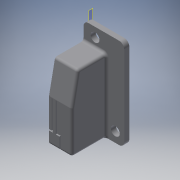
# Autodesk Inventor part: motorBracket_R
Saved by Autodesk Inventor 2016 (Build 200138000, 138)
## iProperties
Created: 2016-09-24
Part Number: motorBracket_R
Material: Generic
Document SubType Name: Modeling
Designer: benja
Density: 1 g/cm^3
Appearance: Default
Author: benja
Autodesk Inventor part; units mm, degrees
ref_plane "YZ Plane" through (0, 0, 0) normal (1, 0, 0) x (0, 1, 0)
ref_plane "XZ Plane" through (0, 0, 0) normal (0, 1, 0) x (-1, 0, 0)
ref_plane "XY Plane" through (0, 0, 0) normal (0, 0, 1) x (1, 0, 0)
ref_plane "Work Plane1" through (29.8157, -13.9206, -3.5875) normal (-1, 0, 0) x (0, -1, 0)
sketch "Sketch1" plane through (29.8157, -13.9206, -3.5875) normal (-1, 0, 0) x (0, -1, 0)
  line L0 (36.0555, 15.1875) -> (19.6981, 15.1875)
  line L1 (7.4278, 14.773) -> (19.5, 17.1875)
  line L2 (19.5, 17.1875) -> (36.0555, 17.1875)
  line L3 (36.0555, 17.1875) -> (36.0555, 15.1875)
  line L4 (0, 0) -> (36.0555, 0) projected
  line L5 (36.0555, 0) -> (36.0555, 1.5875) projected
  line L6 (0, 1.5875) -> (36.0555, 1.5875) projected
  line L7 (0, 0) -> (0, 1.5875) projected
  line L8 (37.8978, 2.9875) -> (37.8978, 4.6582) projected
  line L9 (19.6981, 15.1875) -> (9.4278, 13.1334)
  line L10 (9.4278, 13.1334) -> (9.4278, 2.5875)
  line L11 (9.4278, 2.5875) -> (36.0555, 2.5875)
  line L12 (36.0555, 2.5875) -> (36.0555, 1.5875)
  line L13 (0.4278, 3.5875) -> (7.4278, 3.5875)
  line L14 (7.4278, 3.5875) -> (7.4278, 14.773)
  arc A0 (20.8375, 9.9921) -> (19.4853, 10.9049) centre (20.7278, 11.2875) ccw projected
  arc A1 (19.4853, 10.9049) -> (20.8375, 9.9921) centre (18.0278, 7.2875) ccw projected
  circle A2 centre (15.9478, 12.4775) radius 0.925 projected
  circle A3 centre (12.5278, 5.6875) radius 0.5 projected
  circle A4 centre (30.6778, 13.1375) radius 0.5 projected
  line L15 (13.7278, 4.0975) -> (14.9378, 2.8875) projected
  line L16 (14.9378, 2.8875) -> (21.8778, 2.8875) projected
  line L17 (21.8778, 2.8875) -> (23.7478, 4.7575) projected
  line L18 (23.7478, 4.7575) -> (28.3978, 4.7575) projected
  line L19 (28.3978, 4.7575) -> (28.3978, 11.2875) projected
  line L20 (28.3978, 11.2875) -> (32.9778, 11.2875) projected
  line L21 (32.9778, 11.2875) -> (32.9778, 14.8875) projected
  line L22 (32.9778, 14.8875) -> (19.7278, 14.8875) projected
  line L23 (19.7278, 14.8875) -> (9.7278, 12.8875) projected
  line L24 (9.7278, 6.0975) -> (9.7278, 12.8875) projected
  line L25 (11.7278, 4.0975) -> (9.7278, 6.0975) projected
  line L26 (13.7278, 4.0975) -> (11.7278, 4.0975) projected
  circle A5 centre (27.3778, 12.9875) radius 0.925 projected
  line L27 (36.0555, 1.5875) -> (0, 1.5875)
  line L28 (0.4278, 3.5875) -> (0.4278, 1.5875)
  point P0 (-13.9206, 3.5875)
  dimension "d2" = 2
  dimension "d3" = 0.3
  dimension "d4" = 0.3
  dimension "d5" = 0.3
  dimension "d6" = 0.3
  dimension "d7" = 2
  dimension "d8" = 2
  dimension "d10" = 2
  dimension "d37" = 7
  constraints: 26 end point, 5 perpendicular, 1 collinear, 1 parallel, 1 point on line, 1 vertical
  measures "d2" distance between parallel lines of L2 L0
  measures "d3" distance between parallel lines of L11 L16
  measures "d4" distance between parallel lines of L10 L24
  measures "d5" distance between parallel lines of L23 L9
  measures "d6" distance between parallel lines of L22 L0
  measures "d7" distance between parallel lines of L6 L13
  measures "d8" distance between parallel lines of L14 L10
  measures "d10" distance between parallel lines of L9 L1
  measures "d37" distance between parallel lines of L14 L28
extrude "Extrusion1" add sketch "Sketch1" against normal blind 7.05 contours L0 L9 L10 L11 L12 L6 L28 L13 L14 L1 L2 L3
sketch "Sketch2" plane through (36.8657, -13.9206, -3.5875) normal (1, 0, 0) x (0, 0, -1)
  line L0 (-17.1875, -36.0555) -> (-15.1875, -36.0555) projected
  line L1 (-15.1875, -36.0555) -> (-15.1875, -19.6981) projected
  line L2 (-15.1875, -19.6981) -> (-13.1334, -9.4278) projected
  line L3 (-13.1334, -9.4278) -> (-2.5875, -9.4278) projected
  line L4 (-2.5875, -9.4278) -> (-2.5875, -36.0555) projected
  line L5 (-2.5875, -36.0555) -> (-1.5875, -36.0555) projected
  line L6 (-1.5875, -36.0555) -> (-1.5875, -0.4278) projected
  line L7 (-3.5875, -0.4278) -> (-3.5875, -7.4278) projected
  line L8 (-3.5875, -7.4278) -> (-14.773, -7.4278) projected
  line L9 (-14.773, -7.4278) -> (-17.1875, -19.5) projected
  line L10 (-17.1875, -19.5) -> (-17.1875, -36.0555) projected
  circle A0 centre (-6.6375, -25.4778) radius 0.75 projected
  circle A1 centre (-11.2775, -19.4778) radius 0.75 projected
  circle A2 centre (-11.2775, -19.4778) radius 1.75
  circle A3 centre (-6.6375, -25.4778) radius 1.75
  line L11 (-2.5875, -9.4278) -> (-2.5875, -36.0555) projected
  line L12 (-15.1875, -36.0555) -> (-15.1875, -19.6981) projected
  line L13 (-2.5875, -36.0555) -> (-15.1875, -36.0555)
  line L14 (-1.5875, -0.4278) -> (-3.5875, -0.4278) projected
  point P0 (-3.5875, 13.9206)
  dimension "d13" = 1
  dimension "d14" = 1
  constraints: 2 centre point, 2 end point, 1 horizontal
  measures "d13" radial gap between concentric circles of A1 A2
  measures "d14" radial gap between concentric circles of A0 A3
extrude "Extrusion2" add sketch "Sketch2" along normal blind 0.8 contours L10 L9 L8 L7 L14 L6 L5 L4 L3 L2 L1 L0 | L1 L2 L3 L4 L13
sketch "Sketch3" plane through (37.6657, -13.9206, -3.5875) normal (1, 0, 0) x (0, 0, -1)
  circle A0 centre (-6.6375, -25.4778) radius 1.75 projected
  circle A1 centre (-11.2775, -19.4778) radius 1.75 projected
  line L0 (-17.1875, -36.0555) -> (-1.5875, -36.0555) projected
  line L1 (-1.5875, -36.0555) -> (-1.5875, -0.4278) projected
  line L2 (-3.5875, -0.4278) -> (-3.5875, -7.4278) projected
  line L3 (-3.5875, -7.4278) -> (-14.773, -7.4278) projected
  line L4 (-14.773, -7.4278) -> (-17.1875, -19.5) projected
  line L5 (-17.1875, -19.5) -> (-17.1875, -36.0555) projected
  line L6 (-1.5875, -0.4278) -> (-3.5875, -0.4278) projected
  point P0 (-3.5875, 13.9206)
extrude "Extrusion3" add sketch "Sketch3" along normal blind 1.2 contours A0 | A1 | L5 L4 L3 L2 L6 L1 L0
sketch "Sketch4" plane through (29.8157, -49.9762, -1) normal (0, 0, 1) x (1, 0, 0)
  line L0 (4.5, 22.3278) -> (0.7, 24.9278) projected
  line L1 (6.75, 22.3278) -> (6.75, 16.3278) projected
  line L2 (6.75, 22.3278) -> (0.7, 22.3278) projected
  line L3 (0.7, 26.3278) -> (0.7, 22.3278) projected
  line L4 (0, 26.3278) -> (0.7, 26.3278) projected
  line L5 (0, 16.3278) -> (0, 26.3278) projected
  line L6 (6.75, 16.3278) -> (0, 16.3278) projected
  line L7 (0, 0) -> (0, 26.6278) projected
  line L8 (0, 0) -> (7.05, 0) projected
  line L9 (7.05, 26.6278) -> (7.05, 0) projected
  line L10 (0, 26.6278) -> (7.05, 26.6278) projected
  line L11 (7.05, 26.6278) -> (7.05, 0) projected
  line L12 (7.05, 22.8278) -> (4.6547, 22.8278)
  line L13 (4.6547, 22.8278) -> (1.2, 25.1915)
  line L14 (1.2, 25.1915) -> (1.2, 26.6278)
  line L15 (0, 26.6278) -> (7.05, 26.6278) projected
  point P0 (-29.8157, 49.9762)
  dimension "d19" = 0.5
  dimension "d20" = 0.5
  dimension "d21" = 0.5
  constraints: 6 end point, 2 perpendicular, 2 point on line
  measures "d19" distance between parallel lines of L12 L2
  measures "d20" distance between parallel lines of L0 L13
  measures "d21" distance between parallel lines of L3 L14
extrude "Extrusion4" add sketch "Sketch4" along normal up to next contours L10 L9 L12 L13 L14
sketch "Sketch5" plane through (29.8157, -13.9206, -3.5875) normal (-1, 0, 0) x (0, 0, 1)
  line L0 (2.5875, -9.4278) -> (13.1334, -9.4278) projected
  line L1 (5.6904, -9.4278) -> (2.5875, -12.5306)
  line L2 (2.5875, -36.0555) -> (2.5875, -9.4278) projected
  line L3 (4.0975, -11.7278) -> (6.0975, -9.7278) projected
  point P0 (3.5875, 13.9206)
  dimension "d24" = 0.5
  constraints: 2 end point, 2 point on line, 1 parallel
  measures "d24" distance between parallel lines of L1 L3
extrude "Extrusion5" add sketch "Sketch5" against normal up to next
sketch "Sketch6" plane through (29.8157, -49.9762, -1) normal (0, 0, 1) x (1, 0, 0)
  line L0 (0, 12.3078) -> (0, 7.6578) projected
  line L1 (0, 12.3078) -> (1.8, 12.3078) projected
  line L2 (1.8, 12.3078) -> (1.8, 7.6578) projected
  line L3 (0, 7.6578) -> (1.8, 7.6578) projected
  line L4 (0, 7.9578) -> (0.9, 7.9578)
  line L5 (0.9, 7.9578) -> (0.9, 12.0078)
  line L6 (0.9, 12.0078) -> (0, 12.0078)
  line L7 (0, 0) -> (0, 23.5249) projected
  point P0 (-29.8157, 49.9762)
  dimension "d27" = 0.9
  dimension "d28" = 0.3
  dimension "d29" = 0.3
  constraints: 6 end point, 2 point on line, 1 horizontal, 1 parallel, 1 perpendicular
  measures "d27" distance between parallel lines of L2 L5
  measures "d28" distance between parallel lines of L4 L3
  measures "d29" distance between parallel lines of L1 L6
extrude "Extrusion6" add sketch "Sketch6" along normal blind 1.6 contours L6 L5 L4 L0
sketch "Sketch7" plane through (29.8157, -13.9206, -3.5875) normal (-1, 0, 0) x (0, 0, 1)
  line L0 (4.1875, -24.0478) -> (2.5875, -24.0478) projected
  line L1 (1.5875, -0.4278) -> (1.5875, -36.0555) projected
  line L2 (4.1875, -24.0478) -> (1.5875, -24.0478)
  line L3 (1.5875, -24.0478) -> (1.5875, -28.0978)
  line L4 (1.5875, -28.0978) -> (4.1875, -28.0978)
  line L5 (4.1875, -28.0978) -> (4.1875, -24.0478)
  line L6 (2.5875, -28.0978) -> (4.1875, -28.0978) projected
  point P0 (3.5875, 13.9206)
  point P1 (1.5875, 0)
  constraints: 8 end point, 2 parallel, 1 collinear, 1 horizontal, 1 perpendicular, 1 point on line
extrude "Extrusion7" add sketch "Sketch7" along normal blind 1
fillet "Fillet1" radius 1 1 edges at (28.8157, -39.9934, 0.6)
fillet "Fillet1" radius 0.4 1 edges at (30.7157, -39.9934, 0.6)
sketch "Sketch8" plane through (38.8657, -49.9762, -2) normal (0, 0, -1) x (-1, 0, 0)
  line L0 (9.05, 35.6278) -> (9.05, 12.0078) projected
  line L1 (9.05, 35.6278) -> (0, 35.6278) projected
  line L2 (0, 0) -> (0, 35.6278) projected
  line L3 (9.05, 0) -> (0, 0) projected
  line L4 (9.05, 7.9578) -> (9.05, 0) projected
  line L5 (9.05, 7.9578) -> (10.05, 7.9578) projected
  line L6 (10.05, 12.0078) -> (10.05, 7.9578) projected
  line L7 (9.05, 12.0078) -> (10.05, 12.0078) projected
  line L8 (0, 0) -> (0, 35.6278) projected
  line L9 (0, 0) -> (-7, 0)
  line L10 (-7, 0) -> (-7, 35.6278)
  line L11 (-7, 35.6278) -> (0, 35.6278)
  line L12 (0, 35.6278) -> (0, 0)
  line L13 (9.05, 35.6278) -> (0, 35.6278) projected
  point P0 (38.8657, 49.9762)
  dimension "d38" = 7
  constraints: 8 end point, 2 parallel, 1 collinear, 1 horizontal, 1 perpendicular
  measures "d38" distance of L10.end L11.end
extrude "Extrusion8" add sketch "Sketch8" against normal blind 2 contours L2 L9 L10 L11
sketch "Sketch9" plane through (38.8657, -49.9762, 0) normal (0, 0, 1) x (1, 0, 0)
  line L0 (-9.05, 28.6278) -> (-9.05, 35.6278) projected
  line L1 (-9.05, 28.6278) -> (0, 28.6278) projected
  line L2 (-9.05, 35.6278) -> (7, 35.6278) projected
  line L3 (0, 0) -> (0, 28.6278) projected
  line L4 (0, 0) -> (7, 0) projected
  line L5 (7, 0) -> (7, 35.6278) projected
  line L6 (-9.05, 35.6278) -> (7, 35.6278) construction
  line L7 (-9.05, 28.6278) -> (-9.05, 35.6278) projected
  line L8 (-9.05, 28.6278) -> (0, 28.6278) projected
  line L9 (-9.05, 35.6278) -> (7, 35.6278) projected
  line L10 (0, 0) -> (0, 28.6278) projected
  line L11 (0, 0) -> (7, 0) projected
  line L12 (7, 0) -> (7, 35.6278) projected
  point P0 (-38.8657, 49.9762)
  point P1 (0, 35.6278)
  point P2 (3.5, 4)
  point P3 (-4.5, 32)
  point P4 (3.5, 4)
  point P5 (-4.5, 32)
  dimension "d50" = 4
  dimension "d52" = 28
  dimension "d53" = 8
  dimension "d54" = 3.5
  constraints: 2 coincident
  measures "d50" distance from line of L4 point (3.5, 4)
  measures "d52" vertical distance of point (3.5, 4) point (-4.5, 32)
  measures "d53" horizontal distance of point (3.5, 4) point (-4.5, 32)
  measures "d54" distance from line of L5 point (3.5, 4)
hole "Hole1" at (42.3657, -45.9762, 0) at (34.3657, -17.9762, 0) direction (0, 0, -1) diameter 3.5 end through all
fillet "Fillet3" radius 2 3 edges at (45.8657, -14.3484, -1) (45.8657, -49.9762, -1) (29.8157, -14.3484, -1)
fillet "Fillet4" radius 1 10 edges at (38.8657, -35.6623, 0) (38.8657, -49.9762, 6.8) (34.3407, -49.9762, 13.6) (38.8657, -41.6984, 13.6) (34.3407, -33.4207, 13.6) (38.8657, -27.3845, 12.3928) (34.3407, -21.3484, 11.1855) (38.8657, -21.3484, 5.5928) (34.3407, -21.3484, 0) (29.8157, -49.9762, -1.5)
sketch "Sketch10" plane through (29.8157, -49.9762, -2) normal (0, 0, -1) x (-1, 0, 0)
  circle A0 centre (-12.55, 4) radius 1.75 projected
  circle A1 centre (-4.55, 32) radius 1.75 projected
  arc A2 (0, 33.6278) -> (-2, 35.6278) centre (-2, 33.6278) ccw projected
  line L0 (-2, 35.6278) -> (-14.05, 35.6278) projected
  arc A3 (-14.05, 35.6278) -> (-16.05, 33.6278) centre (-14.05, 33.6278) ccw projected
  line L1 (-16.05, 33.6278) -> (-16.05, 2) projected
  arc A4 (-16.05, 2) -> (-14.05, 0) centre (-14.05, 2) ccw projected
  line L2 (-1, 0) -> (-14.05, 0) projected
  line L3 (0, 7.9578) -> (0, 1) projected
  line L4 (0, 7.9578) -> (1, 7.9578) projected
  line L5 (1, 12.0078) -> (1, 7.9578) projected
  line L6 (0, 12.0078) -> (1, 12.0078) projected
  line L7 (0, 12.0078) -> (-0.9, 12.0078) projected
  line L8 (-0.9, 12.0078) -> (-0.9, 7.9578) projected
  line L9 (-0.9, 7.9578) -> (0, 7.9578) projected
  line L10 (0, 12.0078) -> (0, 23.5249) projected
  line L11 (-1, 0) -> (-7.05, 0) projected
  line L12 (-7.05, 22.8278) -> (-7.05, 0) projected
  line L13 (-7.05, 22.8278) -> (-4.6547, 22.8278) projected
  line L14 (-4.6547, 22.8278) -> (-3.6358, 23.5249) projected
  line L15 (-3.6358, 23.5249) -> (0, 23.5249) projected
  line L16 (0, 7.9578) -> (1, 7.9578) projected
  line L17 (0, 7.9578) -> (-4.05, 7.9578)
  line L18 (-4.05, 7.9578) -> (-4.05, 7.4578)
  line L19 (-4.05, 7.4578) -> (0, 7.4578)
  line L20 (0, 7.4578) -> (0, 7.9578)
  line L21 (-7.05, 6.4578) -> (-2, 6.4578)
  line L22 (-2, 6.4578) -> (-2, 5.9578)
  line L23 (-2, 5.9578) -> (-7.05, 5.9578)
  line L24 (-7.05, 5.9578) -> (-7.05, 6.4578)
  line L25 (1, 12.0078) -> (1, 7.9578) construction
  line L26 (1, 9.9828) -> (-7.05, 9.9828) construction
  line L27 (0, 12.0078) -> (1, 12.0078)
  line L28 (-0.9, 12.0078) -> (0, 12.0078)
  line L29 (0, 12.0078) -> (1, 12.0078)
  line L30 (0, 12.0078) -> (-4.05, 12.0078)
  line L31 (-4.05, 12.0078) -> (-4.05, 12.5078)
  line L32 (-4.05, 12.5078) -> (0, 12.5078)
  line L33 (0, 12.5078) -> (0, 12.0078)
  line L34 (-7.05, 13.5078) -> (-2, 13.5078)
  line L35 (-2, 13.5078) -> (-2, 14.0078)
  line L36 (-2, 14.0078) -> (-7.05, 14.0078)
  line L37 (-7.05, 14.0078) -> (-7.05, 13.5078)
  line L38 (-7.05, 6.4578) -> (-6.55, 6.4578)
  line L39 (-6.55, 6.4578) -> (-6.55, 13.5078)
  line L40 (-6.55, 13.5078) -> (-7.05, 13.5078)
  line L41 (-7.05, 13.5078) -> (-7.05, 6.4578)
  arc A5 (-1, 0) -> (0, 1) centre (-1, 1) ccw projected
  line L42 (0, 1) -> (0, 7.9578) projected
  arc A6 (-1, 0) -> (0, 1) centre (-1, 1) ccw projected
  line L43 (0, 33.6278) -> (0, 12.0078) projected
  point P0 (29.8157, 49.9762)
  dimension "d56" = 3
  dimension "d57" = 2
  dimension "d58" = 0.5
  dimension "d59" = 0.5
  dimension "d60" = 1
  dimension "d63" = 0.5
  constraints: 48 end point, 9 symmetric about line, 6 parallel, 4 perpendicular, 3 horizontal, 3 point on line, 1 midpoint
  measures "d56" distance between parallel lines of L24 L18
  measures "d57" distance between parallel lines of L3 L22
  measures "d58" distance of L17.end L18.end
  measures "d59" distance of L23.end L21.start
  measures "d60" distance between parallel lines of L19 L21
  measures "d63" distance between parallel lines of L12 L39
extrude "Extrusion9" cut sketch "Sketch10" against normal up to surface (1 mm away) contours L10 L7 L30 L31 L32 | L9 L3 L19 L18 L17 | L36 L35 L34 L12 | L34 L39 L21 L12 | L12 L21 L22 L23
sketch "Sketch11" plane through (29.8157, -49.9762, 11.6) normal (0, 0, -1) x (-1, 0, 0)
  line L0 (-6.75, -0.35) -> (-4.42, -0.35) projected
  line L1 (-6.75, 16.3) -> (-6.75, -0.35) projected
  line L2 (-6.75, 16.3) -> (0, 16.3) projected
  line L3 (0, 3.05) -> (0, 16.3) projected
  line L4 (0, 3.05) -> (-4.42, 3.05) projected
  line L5 (-4.42, 3.05) -> (-4.42, -0.35) projected
  line L6 (0, 0) -> (-7.05, 0) projected
  line L7 (0, 0) -> (-4.12, 0)
  line L8 (-4.12, 0) -> (-4.12, 2.75)
  line L9 (-4.12, 2.75) -> (0, 2.75)
  line L10 (0, 2.75) -> (0, 0)
  point P0 (29.8157, 49.9762)
  dimension "d64" = 0.3
  dimension "d65" = 0.3
  constraints: 8 end point, 2 parallel, 1 horizontal, 1 perpendicular
  measures "d64" distance between parallel lines of L5 L8
  measures "d65" distance between parallel lines of L4 L9
extrude "Extrusion10" add sketch "Sketch11" along normal blind 1 contours L6 L8 L9 L10
fillet "Fillet5" radius 1 1 edges at (31.8757, -49.9762, 10.6)
fillet "Fillet5" radius 0.2 1 edges at (31.8757, -47.2262, 10.6)
sketch "Sketch12" plane through (36.8657, -33.6187, 11.6) normal (0, 0, -1) x (-1, 0, 0)
  line L0 (2.93, -13.6075) -> (7.05, -13.6075) projected
  line L1 (7.05, 0) -> (7.05, -13.6075) projected
  line L2 (7.05, 0) -> (0, 0) projected
  line L3 (0, -16.3575) -> (0, 0) projected
  line L4 (2.93, -16.3575) -> (0, -16.3575) projected
  line L5 (2.93, -16.3575) -> (2.93, -13.6075) projected
  line L6 (2.93, -16.3575) -> (0, -16.3575) projected
  line L7 (2.93, -16.3575) -> (2.43, -16.3575)
  line L8 (2.43, -16.3575) -> (2.43, -11.1075)
  line L9 (2.43, -11.1075) -> (2.93, -11.1075)
  line L10 (2.93, -11.1075) -> (2.93, -16.3575)
  line L11 (7.05, 0) -> (0, 0) projected
  line L12 (6.05, 0) -> (5.55, 0)
  line L13 (5.55, 0) -> (5.55, -11.6075)
  line L14 (5.55, -11.6075) -> (6.05, -11.6075)
  line L15 (6.05, -11.6075) -> (6.05, 0)
  line L16 (4.43, 0) -> (3.93, 0)
  line L17 (3.93, 0) -> (3.93, -11.6075)
  line L18 (3.93, -11.6075) -> (4.43, -11.6075)
  line L19 (4.43, -11.6075) -> (4.43, 0)
  line L20 (6.05, -11.6075) -> (7.05, -11.6075)
  line L21 (7.05, -11.6075) -> (7.05, -11.1075)
  line L22 (7.05, -11.1075) -> (6.05, -11.1075)
  line L23 (6.05, -11.1075) -> (6.05, -11.6075)
  line L24 (3.93, -11.6075) -> (2.93, -11.6075)
  line L25 (2.93, -11.6075) -> (2.93, -11.1075)
  line L26 (2.93, -11.1075) -> (3.93, -11.1075)
  line L27 (3.93, -11.1075) -> (3.93, -11.6075)
  point P0 (36.8657, 33.6187)
  dimension "d70" = 1
  dimension "d71" = 0.5
  dimension "d72" = 0.5
  dimension "d73" = 1
  dimension "d74" = 0.5
  dimension "d75" = 2
  dimension "d76" = 0.5
  dimension "d77" = 0.5
  constraints: 40 end point, 10 parallel, 5 horizontal, 5 perpendicular, 2 collinear, 2 point on line
  measures "d70" distance between parallel lines of L1 L15
  measures "d71" distance between parallel lines of L13 L15
  measures "d72" distance between parallel lines of L19 L17
  measures "d73" distance between parallel lines of L10 L17
  measures "d74" distance between parallel lines of L22 L20
  measures "d75" distance between parallel lines of L14 L0
  measures "d76" distance between parallel lines of L26 L24
  measures "d77" distance of L8.end L9.end
extrude "Extrusion11" cut sketch "Sketch12" against normal up to next contours L5 L4 L8 L9 L10 | L10 L26 L17 L24 | L20 L15 L22 L1 | L17 L2 L19 L18 | L14 L13 L2 L15
equation "\"d4\" = d3"
equation "\"d5\" = d4"
equation "\"d6\" = d5"
equation "\"d8\" = d2"
equation "\"d10\" = d2"
equation "\"d59\" = d58"
equation "\"d63\" = d59"
equation "\"d72\" = d71"
equation "\"d73\" = d70"
equation "\"d74\" = d71"
equation "\"d76\" = d71"
equation "\"d77\" = d71"
body "Solid1"
